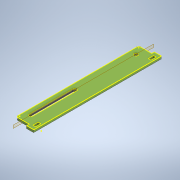
# Autodesk Inventor part: chassis_1_2_up
Saved by Autodesk Inventor 2022 (Build 260153000, 153)
## iProperties
Created: 2023-03-24
Part Number: chassis_1_2_up
Material: 一般
Document SubType Name: Modeling
Designer: Johnny Jou
Density: 1 g/cm^3
Appearance: 預設
Author: Johnny Jou
Autodesk Inventor part; units mm, degrees
ref_plane "YZ Plane" through (0, 0, 0) normal (1, 0, 0) x (0, 1, 0)
ref_plane "XZ Plane" through (0, 0, 0) normal (0, 1, 0) x (-1, 0, 0)
ref_plane "XY Plane" through (0, 0, 0) normal (0, 0, 1) x (1, 0, 0)
sketch "草圖1" plane through (0, 0, 0) normal (0, 1, 0) x (-1, 0, 0)
  line L0 (0, 0) -> (0, -140)
  line L1 (15, -140) -> (15, 0)
  line L2 (6, 0) -> (6, 3)
  line L3 (6, 3) -> (14.1, 3)
  line L4 (14.1, 3) -> (14.1, 0)
  line L5 (15, 0) -> (14.1, 0)
  line L6 (6, 0) -> (0, 0)
  line L7 (6, -140) -> (6, -143)
  line L8 (6, -143) -> (14.1, -143)
  line L9 (14.1, -143) -> (14.1, -140)
  line L10 (0, -140) -> (6, -140)
  line L11 (14.1, -140) -> (15, -140)
  dimension "d1" = 15
  dimension "d2" = 3
  dimension "d3" = 8.1
  dimension "d4" = 6
  dimension "d5" = 3
  dimension "d6" = 140
  dimension "d7" = 6
  dimension "d8" = 8.1
  dimension "d9" = 15
  dimension "d10" = 140
  constraints: 24 end point, 7 parallel, 4 horizontal, 2 perpendicular, 1 coincident
  measures "d1" distance of L1.end L0.start
  measures "d2" distance of L3.end L4.end
  measures "d3" distance of L2.end L3.end
  measures "d4" distance between parallel lines of L0 L2
  measures "d5" distance of L8.end L9.end
  measures "d6" distance of L0.start L0.end
  measures "d7" distance between parallel lines of L0 L7
  measures "d8" distance of L7.end L8.end
  measures "d9" distance between parallel lines of L0 L1
  measures "d10" distance of L1.start L1.end
extrude "擠出1" add sketch "草圖1" along normal blind 3
sketch "草圖2" plane through (0, 3, 0) normal (0, 1, 0) x (1, 0, 0)
  line L0 (-11, 1) -> (-8, 1)
  line L1 (-8, 1) -> (-8, 7)
  line L2 (-8, 7) -> (-11, 7)
  line L3 (-11, 7) -> (-11, 1)
  line L4 (0, 0) -> (0, 140) projected
  line L5 (-6, 0) -> (0, 0) projected
  line L6 (-11, 133) -> (-8, 133)
  line L7 (-8, 133) -> (-8, 139)
  line L8 (-8, 139) -> (-11, 139)
  line L9 (-11, 139) -> (-11, 133)
  line L10 (0, 140) -> (-6, 140) projected
  line L11 (-15, 140) -> (-15, 0) projected
  dimension "d13" = 6
  dimension "d14" = 3
  dimension "d16" = 1
  dimension "d17" = 6
  dimension "d18" = 3
  dimension "d20" = 1
  dimension "d33" = 4
  dimension "d34" = 4
  constraints: 16 end point, 4 parallel, 2 horizontal, 2 perpendicular
  measures "d13" distance of L2.end L0.start
  measures "d14" distance of L1.end L2.end
  measures "d16" distance between parallel lines of L5 L0
  measures "d17" distance of L8.end L6.start
  measures "d18" distance of L6.start L6.end
  measures "d20" distance between parallel lines of L10 L8
  measures "d33" distance between parallel lines of L11 L3
  measures "d34" distance between parallel lines of L11 L9
extrude "擠出2" cut sketch "草圖2" against normal up to surface (3 mm away)
sketch "草圖4" plane through (0, 3, 0) normal (0, 1, 0) x (1, 0, 0)
  line L0 (-27, 0) -> (-15, 0)
  line L1 (-15, 0) -> (-15, 140)
  line L2 (-15, 140) -> (-27, 140)
  line L3 (-29, 138) -> (-29, 2)
  line L4 (-15, 140) -> (-15, 0) projected
  line L5 (0, 140) -> (-6, 140) projected
  line L6 (-6, 0) -> (0, 0) projected
  line L7 (-22, 10) -> (-22, 60) construction
  line L8 (-20, 10) -> (-20, 60)
  line L9 (-24, 60) -> (-24, 10)
  arc A0 (-24, 10) -> (-20, 10) centre (-22, 10) ccw
  arc A1 (-20, 60) -> (-24, 60) centre (-22, 60) ccw
  circle A2 centre (-22, 130) radius 2
  arc A3 (-29, 2) -> (-27, 0) centre (-27, 2) ccw
  arc A4 (-27, 140) -> (-29, 138) centre (-27, 138) ccw
  point P0 (-22, 35)
  dimension "d23" = 14
  dimension "d24" = 4
  dimension "d25" = 50
  dimension "d26" = 5
  dimension "d27" = 10
  dimension "d29" = 2
  dimension "d32" = 10
  constraints: 16 end point, 8 point on circle, 8 tangent, 5 centre point, 3 collinear, 3 parallel, 2 equal radius, 1 horizontal, 1 midpoint, 1 perpendicular, 1 vertical, 1 vertical alignment
  measures "d23" distance between parallel lines of L1 L3
  measures "d24" distance between parallel lines of L8 L9
  measures "d25" distance of L7.end L7.start
  measures "d26" distance between parallel lines of L3 L9
  measures "d27" distance from line of L0 L7.start
  measures "d29" radius of A3
  measures "d32" distance from line of A2.centre L2
extrude "擠出3" add sketch "草圖4" against normal up to surface (3 mm away)
sketch "草圖6" plane through (0, 3, 0) normal (0, 1, 0) x (1, 0, 0)
  circle A0 centre (-22, 130) radius 2 projected
  arc A1 (-24, 10) -> (-20, 10) centre (-22, 10) ccw projected
  line L0 (-24, 10) -> (-24, 60) projected
  arc A2 (-20, 60) -> (-24, 60) centre (-22, 60) ccw projected
  line L1 (-20, 60) -> (-20, 10) projected
  line L2 (-8, 7) -> (-8, 1) projected
  line L3 (-8, 1) -> (-11, 1) projected
  line L4 (-11, 1) -> (-11, 7) projected
  line L5 (-11, 7) -> (-8, 7) projected
  line L6 (-8, 133) -> (-11, 133) projected
  line L7 (-11, 133) -> (-11, 139) projected
  line L8 (-11, 139) -> (-8, 139) projected
  line L9 (-8, 139) -> (-8, 133) projected
  line L10 (0, 0) -> (0, 140) projected
  line L11 (0, 140) -> (-6, 140) projected
  line L12 (-6, 140) -> (-6, 143) projected
  line L13 (-6, 143) -> (-14.1, 143) projected
  line L14 (-14.1, 143) -> (-14.1, 140) projected
  line L15 (-14.1, 140) -> (-27, 140) projected
  arc A3 (-27, 140) -> (-29, 138) centre (-27, 138) ccw projected
  line L16 (-29, 138) -> (-29, 2) projected
  arc A4 (-29, 2) -> (-27, 0) centre (-27, 2) ccw projected
  line L17 (-27, 0) -> (-14.1, 0) projected
  line L18 (-14.1, 0) -> (-14.1, -3) projected
  line L19 (-14.1, -3) -> (-6, -3) projected
  line L20 (-6, -3) -> (-6, 0) projected
  line L21 (-6, 0) -> (0, 0) projected
  line L22 (-6, 140) -> (-6, 143) projected
  line L23 (-6, 0) -> (-6, 140)
  constraints: 2 end point, 1 collinear
extrude "擠出4" cut sketch "草圖6" against normal blind 3 contours L21 L23 L11 L10
sketch "草圖7" plane through (0, 3, 0) normal (0, 1, 0) x (1, 0, 0)
  line L0 (-6, -3) -> (-6, 143) projected
  line L1 (-6, 143) -> (-14.1, 143) projected
  line L2 (-14.1, 143) -> (-14.1, 140) projected
  line L3 (-14.1, 140) -> (-27, 140) projected
  arc A0 (-27, 140) -> (-29, 138) centre (-27, 138) ccw projected
  line L4 (-29, 138) -> (-29, 2) projected
  arc A1 (-29, 2) -> (-27, 0) centre (-27, 2) ccw projected
  line L5 (-27, 0) -> (-14.1, 0) projected
  line L6 (-14.1, 0) -> (-14.1, -3) projected
  line L7 (-14.1, -3) -> (-6, -3) projected
  circle A2 centre (-22, 130) radius 2 projected
  arc A3 (-24, 10) -> (-20, 10) centre (-22, 10) ccw projected
  line L8 (-24, 10) -> (-24, 60) projected
  arc A4 (-20, 60) -> (-24, 60) centre (-22, 60) ccw projected
  line L9 (-20, 60) -> (-20, 10) projected
  line L10 (-8, 7) -> (-8, 1) projected
  line L11 (-8, 1) -> (-11, 1) projected
  line L12 (-11, 1) -> (-11, 7) projected
  line L13 (-11, 7) -> (-8, 7) projected
  line L14 (-8, 133) -> (-11, 133) projected
  line L15 (-11, 133) -> (-11, 139) projected
  line L16 (-11, 139) -> (-8, 139) projected
  line L17 (-8, 139) -> (-8, 133) projected
  point P0 (0, 0)
ref_plane "工作平面1" through (-22, 3, -10) normal (1, 0, 0) x (0, 0, -1)
equation "\"d10\" = d6"
equation "\"d20\" = d16"
